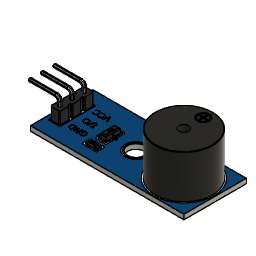
Active (Autodesk Fusion 360 design; units mm, degrees)
Autodesk Fusion 360 part; units mm, degrees
note: some values were not read from the file. Set by a fixed rule: which sketch regions a step uses; which face or edge a step refers to.
(part 1 of 2)
sketch "Sketch1" plane through (0, 0, 0) normal (0, 0, 1) x (1, 0, 0)
  line L0 (16, 6.5) -> (-16, 6.5)
  line L1 (-16, 6.5) -> (-16, -6.5)
  line L2 (-16, -6.5) -> (16, -6.5)
  line L3 (16, -6.5) -> (16, 6.5)
  line L4 (16, 6.5) -> (-16, -6.5) construction
  line L5 (-16, 6.5) -> (16, -6.5) construction
  dimension "d1" = 32
  dimension "d2" = 13
  constraint horizontal L0
  constraint perpendicular L0 L1
  constraint parallel L0 L2
  constraint parallel L1 L3
  constraint coincident L4 origin
  constraint coincident L5 origin
  measures "d1" distance of L1.end L2.end
  measures "d2" distance of L0.end L1.end
extrude "Extrude1" add sketch "Sketch1" along normal blind 1
sketch "Sketch2" plane through (0, 0, 1) normal (0, 0, 1) x (-1, 0, 0)
  line L0 (-16, 6.5) -> (-16, -6.5)
  line L1 (-16, -6.5) -> (16, -6.5)
  line L2 (16, -6.5) -> (16, 6.5)
  line L3 (16, 6.5) -> (-16, 6.5)
  circle A0 centre (-9.5, 0) radius 6
  line L4 (-9.5, 0) -> (-9.5, -6)
  line L5 (-9.5, 0) -> (-15.5, 0)
  circle A1 centre (0.5, 0) radius 1.75
  line L6 (5.25, 1.5) -> (6.5, 1.5)
  line L7 (6.5, 1.5) -> (6.5, -1.5)
  line L8 (6.5, -1.5) -> (5.25, -1.5)
  line L9 (5.25, -1.5) -> (5.25, 1.5)
  line L10 (5.25, 1.5) -> (6.5, -1.5) construction
  line L11 (6.5, 1.5) -> (5.25, -1.5) construction
  line L12 (6.5, 1.5) -> (7.5, 1.5)
  line L13 (7.5, 1.5) -> (7.5, 1)
  line L14 (7.5, 1) -> (6.5, 1)
  line L15 (6.5, 1) -> (6.5, 1.5)
  line L16 (6.5, -1.5) -> (7.5, -1.5)
  line L17 (7.5, -1.5) -> (7.5, -1)
  line L18 (7.5, -1) -> (6.5, -1)
  line L19 (6.5, -1) -> (6.5, -1.5)
  line L20 (5.25, 0.25) -> (4.25, 0.25)
  line L21 (4.25, 0.25) -> (4.25, -0.25)
  line L22 (4.25, -0.25) -> (5.25, -0.25)
  line L23 (5.25, -0.25) -> (5.25, 0.25)
  line L24 (14.325, 2.705) -> (13.675, 2.705)
  line L25 (13.675, 2.705) -> (13.675, 2.055)
  line L26 (13.675, 2.055) -> (14.325, 2.055)
  line L27 (14.325, 2.055) -> (14.325, 2.705)
  line L28 (14.325, 2.705) -> (13.675, 2.055) construction
  line L29 (13.675, 2.705) -> (14.325, 2.055) construction
  line L30 (13.675, -0.485) -> (14.325, -0.485)
  line L31 (14.325, -0.485) -> (14.325, 0.165)
  line L32 (14.325, 0.165) -> (13.675, 0.165)
  line L33 (13.675, 0.165) -> (13.675, -0.485)
  line L34 (13.675, -0.485) -> (14.325, 0.165) construction
  line L35 (14.325, -0.485) -> (13.675, 0.165) construction
  line L36 (13.675, -3.025) -> (14.325, -3.025)
  line L37 (14.325, -3.025) -> (14.325, -2.375)
  line L38 (14.325, -2.375) -> (13.675, -2.375)
  line L39 (13.675, -2.375) -> (13.675, -3.025)
  line L40 (13.675, -3.025) -> (14.325, -2.375) construction
  line L41 (14.325, -3.025) -> (13.675, -2.375) construction
  line L42 (15, 1.38) -> (13, 1.38)
  line L43 (13, 1.38) -> (13, 3.38)
  line L44 (13, 3.38) -> (15, 3.38)
  line L45 (15, 3.38) -> (15, 1.38)
  line L46 (15, 1.38) -> (13, 3.38) construction
  line L47 (13, 1.38) -> (15, 3.38) construction
  line L48 (15, -1.16) -> (13, -1.16)
  line L49 (13, -1.16) -> (13, 0.84)
  line L50 (13, 0.84) -> (15, 0.84)
  line L51 (15, 0.84) -> (15, -1.16)
  line L52 (15, -1.16) -> (13, 0.84) construction
  line L53 (13, -1.16) -> (15, 0.84) construction
  line L54 (13.3, 1.38) -> (13.3, 0.84)
  line L55 (14.7, 1.38) -> (14.7, 0.84)
  line L56 (15, -1.7) -> (13, -1.7)
  line L57 (13, -1.7) -> (13, -3.7)
  line L58 (13, -3.7) -> (15, -3.7)
  line L59 (15, -3.7) -> (15, -1.7)
  line L60 (15, -1.7) -> (13, -3.7) construction
  line L61 (13, -1.7) -> (15, -3.7) construction
  line L62 (13.3, -1.16) -> (13.3, -1.7)
  line L63 (14.7, -1.16) -> (14.7, -1.7)
  circle A2 centre (0.5, 0) radius 2
  circle A3 centre (0.5, 0) radius 2.25
  circle A4 centre (-9.5, 0) radius 6.3
  line L64 (12.8, 1.38) -> (12.8, 3.38)
  line L65 (15.2, 3.38) -> (15.2, 1.38)
  line L66 (12.8, -1.7) -> (12.8, -3.7)
  line L67 (15.2, -3.7) -> (15.2, -1.7)
  line L68 (15.2, 1.38) -> (15.2, -1.7)
  line L69 (12.8, 1.38) -> (12.8, -1.7)
  line L70 (13, 3.58) -> (15, 3.58)
  line L71 (13, -3.9) -> (15, -3.9)
  line L72 (15, -3.9) -> (15.2, -3.9)
  line L73 (15.2, -3.9) -> (15.2, -3.7)
  line L74 (12.8, -3.7) -> (12.8, -3.9)
  line L75 (12.8, -3.9) -> (13, -3.9)
  line L76 (13, 3.58) -> (12.8, 3.58)
  line L77 (12.8, 3.58) -> (12.8, 3.38)
  line L78 (15, 3.58) -> (15.2, 3.58)
  line L79 (15.2, 3.58) -> (15.2, 3.38)
  line L80 (8.4907, 1.5124) -> (11.9345, 1.5124) construction
  line L81 (11.9345, 1.5124) -> (11.9345, 3.2687) construction
  line L82 (11.9345, 3.2687) -> (8.4907, 3.2687) construction
  line L83 (8.4907, 3.2687) -> (8.4907, 1.5124) construction
  line L84 (8.5, -1.25) -> (12.1, -1.25) construction
  line L85 (12.1, -1.25) -> (12.1, 0.95) construction
  line L86 (12.1, 0.95) -> (8.5, 0.95) construction
  line L87 (8.5, 0.95) -> (8.5, -1.25) construction
  line L88 (8.4, -3.85) -> (12.2, -3.85) construction
  line L89 (12.2, -3.85) -> (12.2, -1.65) construction
  line L90 (12.2, -1.65) -> (8.4, -1.65) construction
  line L91 (8.4, -1.65) -> (8.4, -3.85) construction
  line L92 (6.875, 3.125) -> (4.875, 3.125)
  line L93 (4.875, 3.125) -> (4.875, 3.875)
  line L94 (4.875, 3.875) -> (6.875, 3.875)
  line L95 (6.875, 3.875) -> (6.875, 3.125)
  line L96 (6.875, 3.125) -> (4.875, 3.875) construction
  line L97 (4.875, 3.125) -> (6.875, 3.875) construction
  line L98 (4.875, 3.875) -> (5.125, 3.875)
  line L99 (5.125, 3.875) -> (5.125, 3.125)
  line L100 (5.125, 3.125) -> (4.875, 3.125)
  line L101 (4.875, 3.125) -> (4.875, 3.875)
  line L102 (5.125, 3.875) -> (5.375, 3.875)
  line L103 (5.375, 3.875) -> (5.375, 3.125)
  line L104 (5.375, 3.125) -> (5.125, 3.125)
  line L105 (5.125, 3.125) -> (5.125, 3.875)
  line L106 (6.875, 3.875) -> (6.625, 3.875)
  line L107 (6.625, 3.875) -> (6.625, 3.125)
  line L108 (6.625, 3.125) -> (6.875, 3.125)
  line L109 (6.875, 3.125) -> (6.875, 3.875)
  line L110 (6.625, 3.875) -> (6.375, 3.875)
  line L111 (6.375, 3.875) -> (6.375, 3.125)
  line L112 (6.375, 3.125) -> (6.625, 3.125)
  line L113 (6.625, 3.125) -> (6.625, 3.875)
  line L114 (5.375, 3.875) -> (6.375, 3.875)
  line L115 (6.375, 3.875) -> (6.375, 3.8749)
  line L116 (6.375, 3.8749) -> (5.375, 3.8749)
  line L117 (5.375, 3.8749) -> (5.375, 3.875)
  line L118 (5.375, 3.125) -> (6.375, 3.125)
  line L119 (6.375, 3.125) -> (6.375, 3.1251)
  line L120 (6.375, 3.1251) -> (5.375, 3.1251)
  line L121 (5.375, 3.1251) -> (5.375, 3.125)
  line L122 (4.675, 4.075) -> (7.075, 4.075)
  line L123 (7.075, 4.075) -> (7.075, 2.925)
  line L124 (7.075, 2.925) -> (4.675, 2.925)
  line L125 (4.675, 2.925) -> (4.675, 4.075)
  line L126 (7.375, 4.375) -> (7.375, 2.625)
  line L127 (7.375, 2.625) -> (4.375, 2.625)
  line L128 (4.375, 2.625) -> (4.375, 4.375)
  line L129 (4.375, 4.375) -> (7.375, 4.375)
  point P0 (5.875, 0)
  point P1 (5.25, 0)
  point P2 (14, 2.38)
  point P3 (14, -0.16)
  point P4 (14, -2.7)
  point P5 (14, 2.38)
  point P6 (14, -0.16)
  point P7 (14, -2.7)
  point P8 (5.875, 3.5)
  dimension "d5" = 12
  dimension "d17" = 0.5
  dimension "d18" = 0.5
  dimension "d19" = 3.5
  dimension "d20" = 10
  dimension "d22" = 1.25
  dimension "d23" = 3
  dimension "d24" = 6
  dimension "d27" = 1
  dimension "d28" = 0.5
  dimension "d29" = 1
  dimension "d30" = 0.5
  dimension "d31" = 1
  dimension "d32" = 0.5
  dimension "d33" = 0.25
  dimension "d81" = 0.65
  dimension "d82" = 0.65
  dimension "d83" = 0.65
  dimension "d84" = 0.65
  dimension "d85" = 2.54
  dimension "d86" = 0.65
  dimension "d87" = 0.65
  dimension "d88" = 2.54
  dimension "d89" = 3.8
  dimension "d90" = 2
  dimension "d91" = 2
  dimension "d92" = 2
  dimension "d93" = 2
  dimension "d94" = 0.3
  dimension "d95" = 0.3
  dimension "d96" = 2
  dimension "d97" = 2
  dimension "d98" = 0.3
  dimension "d99" = 0.3
  dimension "d132" = 4
  dimension "d133" = 4.5
  dimension "d136" = 12.6
  dimension "d141" = -0.2
  dimension "d142" = -0.2
  dimension "d143" = 0.2
  dimension "d144" = 0.2
  dimension "d145" = -0.2
  dimension "d146" = 0.2
  dimension "d197" = 1.15
  dimension "d198" = 1.15
  dimension "d199" = 1.15
  dimension "d217" = 6.5
  dimension "d218" = 2
  dimension "d219" = 4.12
  dimension "d220" = 6.5
  dimension "d222" = 2
  dimension "d223" = 0.75
  dimension "d224" = 10.125
  dimension "d225" = 3
  dimension "d226" = 0.25
  dimension "d227" = 0.25
  dimension "d228" = 0.25
  dimension "d229" = 0.25
  dimension "d230" = 0.0001
  dimension "d231" = 0.0001
  dimension "d232" = -0.2
  dimension "d233" = -0.5
  text T0 "GND" font "Verdana" height 1.15 align centre middle in box 3.4438 x 1.7563 at (8.4907, 1.5124) x (1, 0) y (0, 1) spacing 1
  text T1 "I/O" font "Verdana" height 1.15 align centre middle in box 3.6 x 2.2 at (8.5, -1.25) x (1, 0) y (0, 1) spacing 1
  text T2 "VCC" font "Verdana" height 1.15 align centre middle in box 3.8 x 2.2 at (8.4, -3.85) x (1, 0) y (0, 1) spacing 1
  constraint coincident A0.centre L4.start
  constraint coincident A0 L4.end
  constraint vertical L4
  constraint coincident A0 L5.end
  constraint perpendicular L4 L5
  constraint horizontal L6
  constraint perpendicular L6 L7
  constraint parallel L6 L8
  constraint parallel L7 L9
  constraint coincident L10 P0
  constraint coincident L11 P0
  constraint horizontal L12
  constraint vertical L13
  constraint horizontal L14
  constraint vertical L15
  constraint horizontal L16
  constraint vertical L17
  constraint horizontal L18
  constraint vertical L19
  constraint horizontal L20
  constraint vertical L21
  constraint horizontal L22
  constraint vertical L23
  constraint coincident L9 L20.start
  constraint midpoint L9 P1
  constraint horizontal L24
  constraint perpendicular L24 L25
  constraint parallel L24 L26
  constraint parallel L25 L27
  constraint coincident L28 P5
  constraint coincident L29 P5
  constraint horizontal L30
  constraint perpendicular L30 L31
  constraint parallel L30 L32
  constraint parallel L31 L33
  constraint coincident L34 P6
  constraint coincident L35 P6
  constraint horizontal L36
  constraint perpendicular L36 L37
  constraint parallel L36 L38
  constraint parallel L37 L39
  constraint coincident L40 P7
  constraint coincident L41 P7
  constraint horizontal L42
  constraint perpendicular L42 L43
  constraint parallel L42 L44
  constraint parallel L43 L45
  constraint coincident L46 P5
  constraint coincident L47 P5
  constraint coincident P5 P2
  constraint horizontal L48
  constraint perpendicular L48 L49
  constraint parallel L48 L50
  constraint parallel L49 L51
  constraint coincident L52 P6
  constraint coincident L53 P6
  constraint coincident P6 P3
  constraint coincident L42 L54.start
  constraint coincident L50 L54.end
  constraint perpendicular L50 L54
  constraint coincident L42 L55.start
  constraint coincident L50 L55.end
  constraint perpendicular L50 L55
  constraint horizontal L56
  constraint perpendicular L56 L57
  constraint parallel L56 L58
  constraint parallel L57 L59
  constraint coincident L60 P7
  constraint coincident L61 P7
  constraint coincident P7 P4
  constraint coincident L48 L62.start
  constraint coincident L56 L62.end
  constraint perpendicular L56 L62
  constraint coincident L48 L63.start
  constraint coincident L56 L63.end
  constraint perpendicular L56 L63
  constraint concentric A1 A2
  constraint concentric A1 A3
  constraint concentric A0 A4
  constraint parallel L71 L72
  constraint parallel L66 L74
  constraint horizontal L76
  constraint horizontal L78
  constraint horizontal L92
  constraint perpendicular L92 L93
  constraint parallel L92 L94
  constraint parallel L93 L95
  constraint coincident L96 P8
  constraint coincident L97 P8
  constraint horizontal L98
  constraint vertical L99
  constraint horizontal L100
  constraint vertical L101
  constraint coincident L92 L99.end
  constraint horizontal L102
  constraint vertical L103
  constraint horizontal L104
  constraint vertical L105
  constraint coincident L92 L103.end
  constraint horizontal L106
  constraint vertical L107
  constraint horizontal L108
  constraint vertical L109
  constraint coincident L92 L107.end
  constraint horizontal L110
  constraint vertical L111
  constraint horizontal L112
  constraint vertical L113
  constraint coincident L92 L111.end
  constraint horizontal L114
  constraint vertical L115
  constraint horizontal L116
  constraint vertical L117
  constraint coincident L111 L115.end
  constraint horizontal L118
  constraint vertical L119
  constraint horizontal L120
  constraint vertical L121
  constraint coincident L111 L119.end
  measures "d5" diameter of A0
  measures "d17" distance of L0 L5.end
  measures "d18" distance of L1 L4.end
  measures "d19" diameter of A1
  measures "d20" distance of A0.centre A1.centre
  measures "d22" distance of L7.end L8.end
  measures "d23" distance of L6.end L7.end
  measures "d24" distance of A1.centre L7
  measures "d27" distance of L6.end L12.end
  measures "d28" distance of L6.end L14.end
  measures "d29" distance of L7.end L16.end
  measures "d30" distance of L7.end L18.end
  measures "d31" distance of L20.start L20.end
  measures "d32" distance of L20.start L22.end
  measures "d33" distance of L20 P1
  measures "d81" distance of L25.end L26.end
  measures "d82" distance of L24.end L25.end
  measures "d83" distance of L31.end L32.end
  measures "d84" distance of L30.end L31.end
  measures "d85" distance of P5 P6
  measures "d86" distance of L37.end L38.end
  measures "d87" distance of L36.end L37.end
  measures "d88" distance of P6 P7
  measures "d89" distance of L1 P7
  measures "d90" distance of L43.end L44.end
  measures "d91" distance of L42.end L43.end
  measures "d92" distance of L49.end L50.end
  measures "d93" distance of L48.end L49.end
  measures "d94" distance of L42.end L54
  measures "d95" distance of L42.start L55
  measures "d96" distance of L57.end L58.end
  measures "d97" distance of L56.end L57.end
  measures "d98" distance of L48.end L62
  measures "d99" distance of L48.start L63
  measures "d132" diameter of A2
  measures "d133" diameter of A3
  measures "d136" diameter of A4
  measures "d217" distance of L3 A1.centre
  measures "d218" distance of L2 P5
  measures "d219" distance of L3 P5
  measures "d220" distance of L1 P0
  measures "d222" distance of L93.end L94.end
  measures "d223" distance of L92.end L93.end
  measures "d224" distance of L2 P8
  measures "d225" distance of L3 P8
  measures "d226" distance of L93.end L98.end
  measures "d227" distance of L98.end L102.end
  measures "d228" distance of L94.end L106.end
  measures "d229" distance of L106.end L110.end
  measures "d230" distance of L102.end L116.end
  measures "d231" distance of L103.end L120.end
extrude "Extrude2" add sketch "Sketch2" along normal blind 9 contours A0 L4 L5 | A0 L4 L5
sketch "Sketch3" plane through (0, 0, 10) normal (0, 0, 1) x (-1, 0, 0)
  circle A0 centre (-9.5, 0) radius 6
  circle A1 centre (-9.5, 0) radius 1
  dimension "d11" = 2
  constraint concentric A0 A1
  measures "d11" diameter of A1
extrude "Extrude3" cut sketch "Sketch3" against normal blind 5 contours A1
extrude "Extrude4" cut sketch "Sketch2" against normal through all contours A1
extrude "Extrude5" add sketch "Sketch2" along normal blind 1 contours L6 L7 L8 L9 L15 L19 L23
extrude "Extrude7" add sketch "Sketch2" along normal blind 0.4001 contours L92 L94 L103 L111 L114 L116 L118 L120
extrude "Extrude8" add sketch "Sketch2" along normal blind 0.4 contours L92 L94 L107 L110 L111 L112 L113 | L92 L94 L99 L102 L103 L104 L105
extrude "Extrude26" add sketch "Sketch2" along normal blind 0.15 contours L92 L94 L95 L106 L107 L108 L109 L113 | L92 L93 L94 L98 L99 L100 L101 L105
fillet "Fillet10" radius 0.05 8 edges at (-5.125, -3.5, 1.4) (-5.25, -3.875, 1.4) (-5.875, -3.8749, 1.4001) (-6.5, -3.875, 1.4) (-6.625, -3.5, 1.4) (-6.5, -3.125, 1.4) (-5.875, -3.1251, 1.4001) (-5.25, -3.125, 1.4)
fillet "Fillet10" radius 0.15 4 edges at (-6.625, -3.5, 1.15) (-6.875, -3.5, 1.15) (-4.875, -3.5, 1.15) (-5.125, -3.5, 1.15)
chamfer "Chamfer1" distance 0.2 distance2 0.2 1 faces at (-6.0833, -0.5, 2)
sketch "Sketch4" plane through (-6.5, 0, 0) normal (-1, 0, 0) x (0, -1, 0)
  line L0 (1.5, 1.8) -> (-1.5, 1.8)
  line L1 (-1.5, 1.8) -> (-1.5, 1)
  line L2 (-1.5, 1) -> (1.5, 1)
  line L3 (1.5, 1) -> (1.5, 1.8)
  line L4 (-1.4, 1) -> (-0.9, 1)
  line L5 (-0.9, 1) -> (-0.9, 1.1)
  line L6 (-0.9, 1.1) -> (-1.4, 1.1)
  line L7 (-1.4, 1.1) -> (-1.4, 1)
  line L8 (0.9, 1) -> (1.4, 1)
  line L9 (1.4, 1) -> (1.4, 1.1)
  line L10 (1.4, 1.1) -> (0.9, 1.1)
  line L11 (0.9, 1.1) -> (0.9, 1)
  dimension "d242" = 0.5
  dimension "d243" = 0.1
  dimension "d244" = 0.5
  dimension "d245" = 0.1
  dimension "d246" = 0.1
  dimension "d247" = 0.1
  constraint horizontal L4
  constraint vertical L5
  constraint horizontal L6
  constraint vertical L7
  constraint coincident L2 L4.start
  constraint horizontal L8
  constraint vertical L9
  constraint horizontal L10
  constraint vertical L11
  constraint coincident L2 L8.start
  measures "d242" distance of L4.start L4.end
  measures "d243" distance of L4.start L6.end
  measures "d244" distance of L8.start L8.end
  measures "d245" distance of L8.start L10.end
  measures "d246" distance of L1 L7
  measures "d247" distance of L3 L9
extrude "Extrude27" add sketch "Sketch4" along normal blind 0.8 contours L2 L8 L9 L10 L11 | L2 L4 L5 L6 L7
sketch "Sketch5" plane through (0, 0, 1.1) normal (0, 0, 1) x (-1, 0, 0)
  line L0 (6.5, -0.9) -> (6.5, -1.4)
  line L1 (6.5, -1.4) -> (7.3, -1.4)
  line L2 (7.3, -1.4) -> (7.3, -0.9)
  line L3 (7.3, -0.9) -> (6.5, -0.9)
  line L4 (6.5, -1.275) -> (6.875, -1.275)
  line L5 (6.875, -1.275) -> (6.875, -1.025)
  line L6 (6.875, -1.025) -> (6.5, -1.025)
  line L7 (6.5, -1.025) -> (6.5, -1.275)
  dimension "d250" = 0.375
  dimension "d251" = 0.25
  dimension "d252" = 0.125
  constraint horizontal L4
  constraint vertical L5
  constraint horizontal L6
  constraint vertical L7
  constraint coincident L0 L4.start
  measures "d250" distance of L4.start L4.end
  measures "d251" distance of L4.start L6.end
  measures "d252" distance of L1 L4
extrude "Extrude28" add sketch "Sketch5" along normal blind 0.2 contours L0 L4 L5 L6 L7
fillet "Fillet11" radius 0.4 1 edges at (-6.5, 1.15, 1.3)
fillet "Fillet11" radius 0.1 1 edges at (-6.875, 1.15, 1.3)
fillet "Fillet12" radius 0.05 6 edges at (-6.5838, 1.275, 1.4543) (-6.8541, 1.275, 1.2763) (-6.875, 1.275, 1.1575) (-6.5838, 1.025, 1.4543) (-6.8541, 1.025, 1.2763) (-6.875, 1.025, 1.1575)
fillet "Fillet13" radius 0.1 2 edges at (-7.3, 1.4, 1.05) (-7.3, 0.9, 1.05)
mirror "Mirror3" about plane through (0, 0, 0) normal (0, 1, 0) of "Extrude28", "Fillet11", "Fillet12", "Fillet13"
fillet "Fillet14" radius 0.1 10 edges at (-6.6625, 1.025, 1.1) (-6.8604, 1.0396, 1.1) (-6.875, 1.15, 1.1) (-6.8604, 1.2604, 1.1) (-6.6625, 1.275, 1.1) (-6.6625, -1.275, 1.1) (-6.8604, -1.2604, 1.1) (-6.875, -1.15, 1.1) (-6.8604, -1.0396, 1.1) (-6.6625, -1.025, 1.1)
sketch "Sketch6" plane through (-5.25, 0, 0) normal (1, 0, 0) x (0, 1, 0)
  line L0 (1.5, 1.8) -> (-1.5, 1.8)
  line L1 (-1.5, 1.8) -> (-1.5, 1)
  line L2 (-1.5, 1) -> (1.5, 1)
  line L3 (1.5, 1) -> (1.5, 1.8)
  line L4 (-0.25, 1) -> (0.25, 1)
  line L5 (0.25, 1) -> (0.25, 1.1)
  line L6 (0.25, 1.1) -> (-0.25, 1.1)
  line L7 (-0.25, 1.1) -> (-0.25, 1)
  dimension "d267" = 0.5
  dimension "d268" = 0.1
  dimension "d269" = 1.25
  constraint horizontal L4
  constraint vertical L5
  constraint horizontal L6
  constraint parallel L5 L7
  constraint coincident L2 L4.start
  measures "d267" distance of L4.start L4.end
  measures "d268" distance of L4.start L6.end
  measures "d269" distance of L3 L5
extrude "Extrude29" add sketch "Sketch6" along normal blind 0.8 contours L2 L4 L5 L6 L7
sketch "Sketch7" plane through (0, 0, 1.1) normal (0, 0, 1) x (-1, 0, 0)
  line L0 (5.25, -0.25) -> (5.25, 0.25)
  line L1 (5.25, 0.25) -> (4.45, 0.25)
  line L2 (4.45, 0.25) -> (4.45, -0.25)
  line L3 (4.45, -0.25) -> (5.25, -0.25)
  line L4 (5.25, 0.125) -> (4.875, 0.125)
  line L5 (4.875, 0.125) -> (4.875, -0.125)
  line L6 (4.875, -0.125) -> (5.25, -0.125)
  line L7 (5.25, -0.125) -> (5.25, 0.125)
  dimension "d272" = 0.375
  dimension "d273" = 0.25
  dimension "d274" = 0.125
  constraint horizontal L4
  constraint vertical L5
  constraint horizontal L6
  constraint vertical L7
  constraint coincident L0 L4.start
  measures "d272" distance of L4.start L4.end
  measures "d273" distance of L4.start L6.end
  measures "d274" distance of L1 L4
extrude "Extrude30" add sketch "Sketch7" along normal blind 0.2 contours L0 L4 L5 L6 L7
fillet "Fillet15" radius 0.4 1 edges at (-5.25, 0, 1.3)
fillet "Fillet15" radius 0.1 3 edges at (-4.875, 0, 1.3) (-4.45, -0.25, 1.05) (-4.45, 0.25, 1.05)
fillet "Fillet16" radius 0.05 6 edges at (-5.1662, -0.125, 1.4543) (-4.8959, -0.125, 1.2763) (-4.875, -0.125, 1.1575) (-5.1662, 0.125, 1.4543) (-4.8959, 0.125, 1.2763) (-4.875, 0.125, 1.1575)
fillet "Fillet17" radius 0.1 5 edges at (-5.0875, 0.125, 1.1) (-4.8896, 0.1104, 1.1) (-4.875, 0, 1.1) (-4.8896, -0.1104, 1.1) (-5.0875, -0.125, 1.1)
fillet "Fillet18" radius 0.1 15 edges at (-4.9, -0.25, 1.1) (-4.4793, -0.2207, 1.1) (-4.45, 0, 1.1) (-4.4793, 0.2207, 1.1) (-4.9, 0.25, 1.1) (-6.85, -1.4, 1.1) (-7.2707, -1.3707, 1.1) (-7.3, -1.15, 1.1) (-7.2707, -0.9293, 1.1) (-6.85, -0.9, 1.1) (-6.85, 0.9, 1.1) (-7.2707, 0.9293, 1.1) (-7.3, 1.15, 1.1) (-7.2707, 1.3707, 1.1) (-6.85, 1.4, 1.1)
extrude "Extrude10" add sketch "Sketch2" along normal blind 2.5 contours L24 L25 L26 L27 | L30 L31 L32 L33 | L36 L37 L38 L39 | L42 L43 L44 L45 | L42 L50 L54 L55 | L48 L49 L50 L51 | L48 L56 L62 L63 | L56 L57 L58 L59
extrude "Extrude11" add sketch "Sketch2" along normal blind 4.5 contours L24 L25 L26 L27 | L30 L31 L32 L33 | L36 L37 L38 L39
sketch "Sketch8" plane through (-14.325, 0, 0) normal (-1, 0, 0) x (0, -1, 0)
  line L0 (-3.025, 3.5) -> (-2.375, 3.5)
  line L1 (-2.375, 3.5) -> (-2.375, 5.5)
  line L2 (-2.375, 5.5) -> (-3.025, 5.5)
  line L3 (-3.025, 5.5) -> (-3.025, 3.5)
  line L4 (-3.025, 5.5) -> (-2.375, 5.5)
  line L5 (-2.375, 5.5) -> (-2.375, 4.85)
  line L6 (-2.375, 4.85) -> (-3.025, 4.85)
  line L7 (-3.025, 4.85) -> (-3.025, 5.5)
  dimension "d104" = 0.65
  dimension "d105" = 0.65
  constraint horizontal L4
  constraint vertical L5
  constraint horizontal L6
  constraint vertical L7
  constraint coincident L2.end L3.start
  measures "d104" distance of L2.end L1.end
  measures "d105" distance of L2.end L6.end
sketch "Sketch9" plane through (-14.325, 0, 0) normal (-1, 0, 0) x (0, -1, 0)
  line L0 (-0.485, 3.5) -> (0.165, 3.5)
  line L1 (0.165, 3.5) -> (0.165, 5.5)
  line L2 (0.165, 5.5) -> (-0.485, 5.5)
  line L3 (-0.485, 5.5) -> (-0.485, 3.5)
  line L4 (-0.485, 5.5) -> (0.165, 5.5)
  line L5 (0.165, 5.5) -> (0.165, 4.85)
  line L6 (0.165, 4.85) -> (-0.485, 4.85)
  line L7 (-0.485, 4.85) -> (-0.485, 5.5)
  dimension "d108" = 0.65
  dimension "d109" = 0.65
  constraint horizontal L4
  constraint vertical L5
  constraint horizontal L6
  constraint vertical L7
  constraint coincident L2.end L3.start
  measures "d108" distance of L2.end L1.end
  measures "d109" distance of L2.end L6.end
sketch "Sketch10" plane through (-14.325, 0, 0) normal (-1, 0, 0) x (0, -1, 0)
  line L0 (2.055, 3.5) -> (2.705, 3.5)
  line L1 (2.705, 3.5) -> (2.705, 5.5)
  line L2 (2.705, 5.5) -> (2.055, 5.5)
  line L3 (2.055, 5.5) -> (2.055, 3.5)
  line L4 (2.055, 5.5) -> (2.705, 5.5)
  line L5 (2.705, 5.5) -> (2.705, 4.85)
  line L6 (2.705, 4.85) -> (2.055, 4.85)
  line L7 (2.055, 4.85) -> (2.055, 5.5)
  dimension "d110" = 0.65
  dimension "d111" = 0.65
  constraint horizontal L4
  constraint vertical L5
  constraint horizontal L6
  constraint vertical L7
  constraint coincident L2.end L3.start
  measures "d110" distance of L2.end L1.end
  measures "d111" distance of L2.end L6.end
extrude "Extrude13" add sketch "Sketch8" sketch "Sketch10" sketch "Sketch9" along normal blind 6 contours L1 L2 L3 L4 L5 L6 L7 of sketch 2 contours L1 L2 L3 L4 L5 L6 L7 of sketch 3 contours L1 L2 L3 L4 L5 L6 L7
fillet "Fillet1" radius 0.1 1 edges at (15.094, 2.1697, 10)
fillet "Fillet6" radius 0.2 12 edges at (-15, 3.7, 2.25) (-13, 3.7, 2.25) (-13, 1.7, 2.25) (-13, -1.38, 2.25) (-13, -0.84, 2.25) (-13, -3.38, 2.25) (-15, -3.38, 2.25) (-15, -1.38, 2.25) (-15, -0.84, 2.25) (-15, 1.16, 2.25) (-15, 1.7, 2.25) (-13, 1.16, 2.25)
fillet "Fillet7" radius 1 3 edges at (-13.675, 2.7, 5.5) (-13.675, 0.16, 5.5) (-13.675, -2.38, 5.5)
fillet "Fillet8" radius 0.5 3 edges at (-14.325, 2.7, 4.85) (-14.325, 0.16, 4.85) (-14.325, -2.38, 4.85)
fillet "Fillet9" radius 0.2 48 edges at (-13.675, 0.485, 4) (-13.9679, 0.485, 5.2071) (-17.5, 0.485, 5.5) (-14.325, 2.375, 3.925) (-14.4714, 2.375, 4.7036) (-17.575, 2.375, 4.85) (-13.675, -0.165, 4) (-13.9679, -0.165, 5.2071) (-17.5, -0.165, 5.5) (-14.325, -2.055, 3.925) (-14.4714, -2.055, 4.7036) (-17.575, -2.055, 4.85) (-20.325, -2.38, 5.5) (-14.325, -0.165, 3.925) (-14.4714, -0.165, 4.7036) (-17.575, -0.165, 4.85) (-13.675, -2.055, 4) (-13.9679, -2.055, 5.2071) (-17.5, -2.055, 5.5) (-20.325, 3.025, 5.175) (-20.325, 2.375, 5.175) (-20.325, -2.705, 5.175) (-20.325, 0.485, 5.175) (-13.675, 3.025, 4) (-13.9679, 3.025, 5.2071) (-17.5, 3.025, 5.5) (-17.5, -2.705, 5.5) (-13.9679, -2.705, 5.2071) (-13.675, -2.705, 4) (-17.575, 3.025, 4.85) (-14.4714, 3.025, 4.7036) (-14.325, 3.025, 3.925) (-20.325, 0.16, 5.5) (-20.325, -2.38, 4.85) (-20.325, 2.7, 4.85) (-14.325, 0.485, 3.925) (-14.4714, 0.485, 4.7036) (-17.575, 0.485, 4.85) (-20.325, -2.055, 5.175) (-20.325, 2.7, 5.5) (-20.325, 0.16, 4.85) (-13.675, 2.375, 4) (-13.9679, 2.375, 5.2071) (-17.5, 2.375, 5.5) (-14.325, -2.705, 3.925) (-14.4714, -2.705, 4.7036) (-17.575, -2.705, 4.85) (-20.325, -0.165, 5.175)
sketch "Sketch11" plane through (0, 1.5, 0) normal (0, 1, 0) x (-1, 0, 0)
  line L0 (6.5, 1) -> (6.5, 1.8)
  line L1 (5.25, 1.8) -> (5.25, 1)
  line L2 (5.25, 1) -> (6.5, 1)
  line L3 (6.5, 1.8) -> (5.25, 1.8)
extrude "Extrude14" add sketch "Sketch2" along normal blind 0.01 contours A3 | A4 | L64 L65 L66 L67 L68 L69 L70 L71 L72 L73 L74 L75 L76 L77 L78 L79
sketch "Sketch12" plane through (0, 0, 0) normal (0, 0, -1) x (1, 0, 0)
  circle A0 centre (-0.5, 0) radius 1.75
  line L0 (16, -6.5) -> (16, 6.5)
  line L1 (16, 6.5) -> (-16, 6.5)
  line L2 (-16, 6.5) -> (-16, -6.5)
  line L3 (-16, -6.5) -> (16, -6.5)
  circle A1 centre (-14, -2.7) radius 1
  circle A2 centre (-14, -0.16) radius 1
  circle A3 centre (-14, -2.7) radius 1.15
  circle A4 centre (-14, -0.16) radius 1.15
  circle A5 centre (-14, 2.38) radius 1.15
  circle A6 centre (-14, 2.38) radius 1
  line L4 (-14.325, -2.375) -> (-13.675, -2.375)
  line L5 (-13.675, -2.375) -> (-13.675, -3.025)
  line L6 (-13.675, -3.025) -> (-14.325, -3.025)
  line L7 (-14.325, -3.025) -> (-14.325, -2.375)
  line L8 (-14.325, -2.375) -> (-13.675, -3.025) construction
  line L9 (-13.675, -2.375) -> (-14.325, -3.025) construction
  line L10 (-14.325, 0.165) -> (-13.675, 0.165)
  line L11 (-13.675, 0.165) -> (-13.675, -0.485)
  line L12 (-13.675, -0.485) -> (-14.325, -0.485)
  line L13 (-14.325, -0.485) -> (-14.325, 0.165)
  line L14 (-14.325, 0.165) -> (-13.675, -0.485) construction
  line L15 (-13.675, 0.165) -> (-14.325, -0.485) construction
  line L16 (-14.325, 2.705) -> (-13.675, 2.705)
  line L17 (-13.675, 2.705) -> (-13.675, 2.055)
  line L18 (-13.675, 2.055) -> (-14.325, 2.055)
  line L19 (-14.325, 2.055) -> (-14.325, 2.705)
  line L20 (-14.325, 2.705) -> (-13.675, 2.055) construction
  line L21 (-13.675, 2.705) -> (-14.325, 2.055) construction
  point P0 (-14, -0.16)
  point P1 (-14, -2.7)
  point P2 (-14, 2.38)
  point P3 (-14, -2.7)
  point P4 (-14, -0.16)
  point P5 (-14, 2.38)
  dimension "d149" = 2
  dimension "d150" = 2
  dimension "d171" = 2.3
  dimension "d172" = 2.3
  dimension "d182" = 2.3
  dimension "d183" = 2
  dimension "d202" = 0.65
  dimension "d203" = 0.65
  dimension "d204" = 0.65
  dimension "d205" = 0.65
  dimension "d206" = 0.65
  dimension "d207" = 0.65
  dimension "d215" = 2
  dimension "d216" = 2.54
  constraint coincident P3 P1
  constraint coincident P4 P0
  constraint coincident P5 P2
  constraint concentric A5 A6
  constraint horizontal L4
  constraint perpendicular L4 L5
  constraint parallel L4 L6
  constraint parallel L5 L7
  constraint coincident L8 P3
  constraint coincident L9 P3
  constraint horizontal L10
  constraint perpendicular L10 L11
  constraint parallel L10 L12
  constraint parallel L11 L13
  constraint coincident L14 P4
  constraint coincident L15 P4
  constraint horizontal L16
  constraint perpendicular L16 L17
  constraint parallel L16 L18
  constraint parallel L17 L19
  constraint coincident L20 P5
  constraint coincident L21 P5
  measures "d149" diameter of A1
  measures "d150" diameter of A2
  measures "d171" diameter of A3
  measures "d172" diameter of A4
  measures "d182" diameter of A5
  measures "d183" diameter of A6
  measures "d202" distance of L5.end L6.end
  measures "d203" distance of L4.end L5.end
  measures "d204" distance of L11.end L12.end
  measures "d205" distance of L10.end L11.end
  measures "d206" distance of L17.end L18.end
  measures "d207" distance of L16.end L17.end
  measures "d215" distance of L2 P4
  measures "d216" distance of P3 P4
extrude "Extrude15" add sketch "Sketch12" along normal blind 1.5 contours L4 L5 L6 L7 | L10 L11 L12 L13 | L16 L17 L18 L19
loft "Loft1" add profiles "Sketch12" section 1 face at (-14.1083, -2.4883, -1.5) section 2 contours A6
loft "Loft2" add profiles "Sketch12" section 1 contours A2 | L10 L11 L12 L13 section 2 face at (-13.8917, 0.2683, -1.5)
loft "Loft6" add profiles "Sketch12" section 1 face at (-14.1083, 2.5917, -1.5) section 2 contours A1
sketch "Sketch13" plane through (0, 0, 0) normal (0, 0, -1) x (1, 0, 0)
  circle A0 centre (-0.5, 0) radius 1.75
  line L0 (16, -6.5) -> (16, 6.5)
  line L1 (16, 6.5) -> (-16, 6.5)
  line L2 (-16, 6.5) -> (-16, -6.5)
  line L3 (-16, -6.5) -> (16, -6.5)
  circle A1 centre (9.5, -3.5) radius 1
  circle A2 centre (9.5, -3.5) radius 0.35
  line L4 (10.5, 2.5) -> (8.5, 2.5)
  line L5 (8.5, 2.5) -> (8.5, 4.5)
  line L6 (8.5, 4.5) -> (10.5, 4.5)
  line L7 (10.5, 4.5) -> (10.5, 2.5)
  line L8 (10.5, 2.5) -> (8.5, 4.5) construction
  line L9 (8.5, 2.5) -> (10.5, 4.5) construction
  line L10 (9.85, 3.15) -> (9.15, 3.15)
  line L11 (9.15, 3.15) -> (9.15, 3.85)
  line L12 (9.15, 3.85) -> (9.85, 3.85)
  line L13 (9.85, 3.85) -> (9.85, 3.15)
  line L14 (9.85, 3.15) -> (9.15, 3.85) construction
  line L15 (9.15, 3.15) -> (9.85, 3.85) construction
  line L16 (10.75, 2.25) -> (8.25, 2.25)
  line L17 (8.25, 2.25) -> (8.25, 4.75)
  line L18 (8.25, 4.75) -> (10.75, 4.75)
  line L19 (10.75, 4.75) -> (10.75, 2.25)
  line L20 (10.75, 2.25) -> (8.25, 4.75) construction
  line L21 (8.25, 2.25) -> (10.75, 4.75) construction
  circle A3 centre (9.5, -3.5) radius 1.2
  spline S0 degree 3 poles (-13.2929, -0.8671) (-13.4758, -1.05) (-13.7318, -1.1575) (-13.9904, -1.16) (-14.2554, -1.1625) (-14.5197, -1.0545) (-14.7071, -0.8671) knots -1 -1 -1 -1 -0.506107 -0.506107 -0.506107 0 0 0 0
  spline S1 degree 3 poles (-14.7071, -0.8671) (-14.89, -0.6842) (-14.9975, -0.4282) (-15, -0.1696) (-15.0025, 0.0954) (-14.8945, 0.3597) (-14.7071, 0.5471) knots -1 -1 -1 -1 -0.506107 -0.506107 -0.506107 0 0 0 0
  spline S2 degree 3 poles (-14.7071, 0.5471) (-14.5242, 0.73) (-14.2682, 0.8375) (-14.0096, 0.84) (-13.7446, 0.8425) (-13.4803, 0.7345) (-13.2929, 0.5471) knots -1 -1 -1 -1 -0.506107 -0.506107 -0.506107 0 0 0 0
  spline S3 degree 3 poles (-13.2929, 0.5471) (-13.11, 0.3642) (-13.0025, 0.1082) (-13, -0.1504) (-12.9975, -0.4154) (-13.1055, -0.6797) (-13.2929, -0.8671) knots -1 -1 -1 -1 -0.506107 -0.506107 -0.506107 0 0 0 0
  spline S4 degree 3 poles (-14.7071, 1.6729) (-14.8945, 1.8603) (-15.0025, 2.1246) (-15, 2.3896) (-14.9975, 2.6482) (-14.89, 2.9042) (-14.7071, 3.0871) knots 0 0 0 0 0.506107 0.506107 0.506107 1 1 1 1
  spline S5 degree 3 poles (-14.7071, 3.0871) (-14.5197, 3.2745) (-14.2554, 3.3825) (-13.9904, 3.38) (-13.7318, 3.3775) (-13.4758, 3.27) (-13.2929, 3.0871) knots 0 0 0 0 0.506107 0.506107 0.506107 1 1 1 1
  spline S6 degree 3 poles (-13.2929, 3.0871) (-13.1055, 2.8997) (-12.9975, 2.6354) (-13, 2.3704) (-13.0025, 2.1118) (-13.11, 1.8558) (-13.2929, 1.6729) knots 0 0 0 0 0.506107 0.506107 0.506107 1 1 1 1
  spline S7 degree 3 poles (-14.7071, -3.4071) (-14.8945, -3.2197) (-15.0025, -2.9554) (-15, -2.6904) (-14.9975, -2.4318) (-14.89, -2.1758) (-14.7071, -1.9929) knots 0 0 0 0 0.506107 0.506107 0.506107 1 1 1 1
  spline S8 degree 3 poles (-14.7071, -1.9929) (-14.5197, -1.8055) (-14.2554, -1.6975) (-13.9904, -1.7) (-13.7318, -1.7025) (-13.4758, -1.81) (-13.2929, -1.9929) knots 0 0 0 0 0.506107 0.506107 0.506107 1 1 1 1
  spline S9 degree 3 poles (-13.2929, -1.9929) (-13.1055, -2.1803) (-12.9975, -2.4446) (-13, -2.7096) (-13.0025, -2.9682) (-13.11, -3.2242) (-13.2929, -3.4071) knots 0 0 0 0 0.506107 0.506107 0.506107 1 1 1 1
  spline S10 degree 3 poles (-13.2929, -3.4071) (-13.4803, -3.5945) (-13.7446, -3.7025) (-14.0096, -3.7) (-14.2682, -3.6975) (-14.5242, -3.59) (-14.7071, -3.4071) knots 0 0 0 0 0.506107 0.506107 0.506107 1 1 1 1
  spline S11 degree 3 poles (-13.2929, 1.6729) (-13.4803, 1.4855) (-13.7446, 1.3775) (-14.0096, 1.38) (-14.2682, 1.3825) (-14.5242, 1.49) (-14.7071, 1.6729) knots 0 0 0 0 0.506107 0.506107 0.506107 1 1 1 1
  point P0 (9.5, 3.5)
  point P1 (9.5, 3.5)
  point P2 (9.5, 3.5)
  dimension "d159" = 2
  dimension "d160" = 3
  dimension "d161" = 6.5
  dimension "d162" = 0.7
  dimension "d163" = 2
  dimension "d164" = 2
  dimension "d165" = 6.5
  dimension "d166" = 3
  dimension "d167" = 0.7
  dimension "d168" = 0.7
  dimension "d173" = 2.5
  dimension "d174" = 2.5
  dimension "d175" = 2.4
  constraint concentric A1 A2
  constraint horizontal L4
  constraint perpendicular L4 L5
  constraint parallel L4 L6
  constraint parallel L5 L7
  constraint coincident L8 P2
  constraint coincident L9 P2
  constraint horizontal L10
  constraint perpendicular L10 L11
  constraint parallel L10 L12
  constraint parallel L11 L13
  constraint coincident L14 P2
  constraint coincident L15 P2
  constraint coincident P2 P1
  constraint horizontal L16
  constraint perpendicular L16 L17
  constraint parallel L16 L18
  constraint parallel L17 L19
  constraint coincident L20 P2
  constraint coincident L21 P2
  constraint concentric A1 A3
  measures "d159" diameter of A1
  measures "d160" distance of L3 A1.centre
  measures "d161" distance of L0 A1.centre
  measures "d162" diameter of A2
  measures "d163" distance of L5.end L6.end
  measures "d164" distance of L4.end L5.end
  measures "d165" distance of L0 P2
  measures "d166" distance of L1 P2
  measures "d167" distance of L11.end L12.end
  measures "d168" distance of L10.end L11.end
  measures "d173" distance of L17.end L18.end
  measures "d174" distance of L16.end L17.end
  measures "d175" diameter of A3
extrude "Extrude17" add sketch "Sketch13" along normal blind 1 contours A2 | L10 L11 L12 L13
loft "Loft3" add profiles "Sketch13" section 1 contours L4 L5 L6 L7 section 2 face at (9.6167, -3.3833, -1)
loft "Loft4" add profiles "Sketch13" section 1 contours A1 section 2 face at (9.3453, 3.5353, -1)
extrude "Extrude18" cut sketch "Sketch13" sketch "Sketch12" against normal blind 0.2 contours L16 L17 L18 L19 | A3 of sketch 2 contours A3 | A4 | A5
sketch "Sketch14" plane through (0, 0, 10) normal (0, 0, 1) x (-1, 0, 0)
  circle A0 centre (-9.5, 0) radius 1
  circle A1 centre (-9.5, 0) radius 5.9
  circle A2 centre (-9.5575, -3.9997) radius 1
  circle A3 centre (-9.5575, -3.9997) radius 1.25
  line L0 (-9.6825, -3.1997) -> (-9.4325, -3.1997)
  line L1 (-9.4325, -3.1997) -> (-9.4325, -4.7997)
  line L2 (-9.4325, -4.7997) -> (-9.6825, -4.7997)
  line L3 (-9.6825, -4.7997) -> (-9.6825, -3.1997)
  line L4 (-9.6825, -3.1997) -> (-9.4325, -4.7997) construction
  line L5 (-9.4325, -3.1997) -> (-9.6825, -4.7997) construction
  line L6 (-10.3575, -4.1247) -> (-8.7575, -4.1247)
  line L7 (-8.7575, -4.1247) -> (-8.7575, -3.8747)
  line L8 (-8.7575, -3.8747) -> (-10.3575, -3.8747)
  line L9 (-10.3575, -3.8747) -> (-10.3575, -4.1247)
  line L10 (-10.3575, -4.1247) -> (-8.7575, -3.8747) construction
  line L11 (-8.7575, -4.1247) -> (-10.3575, -3.8747) construction
  point P0 (-9.5575, -5.8997)
  point P1 (-9.5575, -3.9997)
  point P2 (-9.5575, -3.9997)
  dimension "d187" = 2
  dimension "d188" = 1.9
  dimension "d190" = 2.5
  dimension "d191" = 0.25
  dimension "d192" = 1.6
  dimension "d193" = 1.6
  dimension "d194" = 0.25
  constraint coincident A1 P0
  constraint concentric A2 A3
  constraint horizontal L0
  constraint perpendicular L0 L1
  constraint parallel L0 L2
  constraint parallel L1 L3
  constraint coincident L4 P2
  constraint coincident L5 P2
  constraint coincident P2 P1
  constraint horizontal L6
  constraint perpendicular L6 L7
  constraint parallel L6 L8
  constraint parallel L7 L9
  constraint coincident L10 P2
  constraint coincident L11 P2
  measures "d187" diameter of A2
  measures "d188" distance of P1 P0
  measures "d190" diameter of A3
  measures "d191" distance of L1.end L2.end
  measures "d192" distance of L0.end L1.end
  measures "d193" distance of L7.end L8.end
  measures "d194" distance of L6.end L7.end
extrude "Extrude21" cut sketch "Sketch14" against normal blind 0.05 contours A3 | L0 L1 L3 L8 | L1 L3 L6 L8 | L3 L6 L8 L9 | L1 L6 L7 L8 | L1 L2 L3 L6
extrude "Extrude22" add sketch "Sketch2" along normal blind 0.005 text T0 T1 T2
sketch "Sketch15" plane through (0, 0, 1.4001) normal (0, 0, 1) x (-1, 0, 0)
  line L0 (5.375, 3.1751) -> (6.375, 3.1751)
  line L1 (6.375, 3.1751) -> (6.375, 3.8249)
  line L2 (6.375, 3.8249) -> (5.375, 3.8249)
  line L3 (5.375, 3.8249) -> (5.375, 3.1751)
  line L4 (5.375, 3.1751) -> (6.375, 3.1751) construction
  line L5 (6.375, 3.1751) -> (6.375, 3.8249) construction
  line L6 (6.375, 3.8249) -> (5.375, 3.8249) construction
  line L7 (5.375, 3.8249) -> (5.375, 3.1751) construction
  dimension "d287" = 0.35
  text T0 "102" font "Verdana" height 0.35 align centre middle in box 1 x 0.6498 at (5.375, 3.1751) x (1, 0) y (0, 1) spacing 1
  constraint coincident L0.end
  constraint coincident L2.end
extrude "Extrude31" add sketch "Sketch15" along normal blind 0.001 text T0
sketch "Sketch16" plane through (0, 0, 2) normal (0, 0, 1) x (-1, 0, 0)
  line L0 (6.3, 1.3) -> (5.45, 1.3)
  line L1 (5.45, 1.3) -> (5.45, -1.3)
  line L2 (5.45, -1.3) -> (6.3, -1.3)
  line L3 (6.3, -1.3) -> (6.3, 1.3)
  line L4 (6.3, -1.3) -> (6.3, 1.3) construction
  line L5 (6.3, 1.3) -> (5.45, 1.3) construction
  line L6 (5.45, 1.3) -> (5.45, -1.3) construction
  line L7 (5.45, -1.3) -> (6.3, -1.3) construction
  dimension "d290" = 0.5
  text T0 "2TY" font "Verdana" height 0.5 align centre middle in box 2.6 x 0.85 at (6.3, -1.3) x (0, 1) y (-1, 0) spacing 1
  constraint coincident L0.start
  constraint coincident L1.end
extrude "Extrude32" add sketch "Sketch16" along normal blind 0.001 text T0
extrude "Extrude34" cut 3 faces at (-15.1333, -0.1067, 1.01) (-2.6508, 0.2111, 1.01) (15.6765, 0.313, 1.01) along direction (0, 0, -1) blind 0.009
extrude "Extrude35" cut 8 faces at (-9.4636, -2.1847, 1.005) (-10.611, -2.2692, 1.005) (-11.0154, -2.5385, 1.005) (-9.335, 0.3025, 1.005) (-10.0767, 0.0021, 1.005) (-10.5592, 0.2155, 1.005) (-9.0102, 2.8956, 1.005) (-9.9222, 2.9387, 1.005) along direction (0, 0, -1) blind 0.004